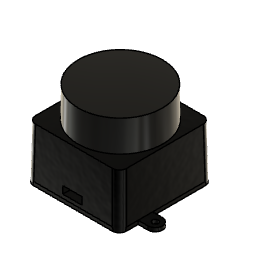
LD19激光雷达 v2 (Autodesk Fusion 360 design; units mm, degrees)
Autodesk Fusion 360 part; units mm, degrees
sketch "草图1" plane through (0, 0, 0) normal (0, 0, 1) x (1, 0, 0)
  line L0 (0, 0) -> (38.59, 0)
  line L1 (38.59, 0) -> (38.59, 38.59)
  line L2 (38.59, 38.59) -> (0, 38.59)
  line L3 (0, 38.59) -> (0, 0)
  line L4 (19.295, 40.7359) -> (19.295, -30)
  circle A0 centre (-4.105, 10.78) radius 1.25
  circle A1 centre (-4.105, 10.78) radius 3
  circle A2 centre (42.695, 10.78) radius 1.25
  circle A3 centre (42.695, 10.78) radius 3
  circle A4 centre (19.3, 42.7) radius 1.25
  circle A5 centre (19.3, 42.7) radius 3
  line L5 (16.3, 38.59) -> (22.3, 38.59)
  line L6 (22.3, 38.59) -> (22.3, 42.7)
  line L7 (16.3, 42.7) -> (16.3, 38.59)
  line L8 (38.59, 13.78) -> (42.695, 13.78)
  line L9 (42.695, 7.78) -> (38.59, 7.78)
  line L10 (38.59, 7.78) -> (38.59, 13.78)
  line L11 (0, 13.78) -> (-4.105, 13.78)
  line L12 (-4.105, 7.78) -> (0, 7.78)
  line L13 (0, 7.78) -> (0, 13.78)
  dimension "d1" = 38.59
  dimension "d2" = 38.59
  dimension "d3" = 2.5
  dimension "d4" = 6
  dimension "d5" = 46.8
  dimension "d6" = 27.81
  dimension "d7" = 2.5
  dimension "d8" = 6
  dimension "d9" = 19.29
  dimension "d10" = 31.92
  constraint horizontal L0
  constraint vertical L1
  constraint horizontal L2
  constraint vertical L3
  constraint coincident L0.start L3.end
  constraint perpendicular L2 L4
  constraint concentric A0 A1
  constraint symmetric L4 A0 A2
  constraint symmetric L4 A1 A3
  constraint concentric A4 A5
  constraint horizontal L5
  constraint vertical L6
  constraint vertical L7
  constraint coincident L2 L5.start
  constraint tangent A5 L7
  constraint tangent A5 L6
  constraint coincident A5 L6.end
  constraint coincident A5 L7.start
  constraint horizontal L8
  constraint horizontal L9
  constraint vertical L10
  constraint coincident L1 L8.start
  constraint tangent A3 L8
  constraint tangent A3 L9
  constraint coincident A3 L8.end
  constraint coincident A3 L9.start
  constraint horizontal L11
  constraint horizontal L12
  constraint vertical L13
  constraint coincident L3 L11.start
  constraint tangent A1 L11
  constraint tangent A1 L12
  constraint coincident A1 L11.end
  constraint coincident A1 L12.start
  measures "d1" distance of L1.end L2.end
  measures "d2" distance of L0.start L2.end
  measures "d3" diameter of A0
  measures "d4" diameter of A1
  measures "d5" distance of A0.centre A2.centre
  measures "d6" distance of L2 A2.centre
  measures "d7" diameter of A4
  measures "d8" diameter of A5
  measures "d9" distance of L1 A4.centre
  measures "d10" vertical distance of A2.centre A4.centre
extrude "拉伸1" add sketch "草图1" along normal blind 1.5 makes body 1
sketch "草图2" plane through (0, 0, 1.5) normal (0, 0, 1) x (-1, 0, 0)
  circle A0 centre (-42.695, -10.78) radius 1.25
  circle A1 centre (4.105, -10.78) radius 1.25
  circle A2 centre (-19.3, -42.7) radius 1.25
  line L0 (-38.59, -13.78) -> (-38.59, -38.59)
  line L1 (-38.59, -38.59) -> (-22.3, -38.59)
  line L2 (-22.3, -38.59) -> (-22.3, -42.7)
  arc A3 (-22.3, -42.7) -> (-16.3, -42.7) centre (-19.3, -42.7) ccw
  line L3 (-16.3, -42.7) -> (-16.3, -38.59)
  line L4 (-16.3, -38.59) -> (0, -38.59)
  line L5 (0, -38.59) -> (0, -13.78)
  line L6 (0, -13.78) -> (4.105, -13.78)
  arc A4 (4.105, -13.78) -> (4.105, -7.78) centre (4.105, -10.78) ccw
  line L7 (4.105, -7.78) -> (0, -7.78)
  line L8 (0, -7.78) -> (0, 0)
  line L9 (0, 0) -> (-38.59, 0)
  line L10 (-38.59, 0) -> (-38.59, -7.78)
  line L11 (-38.59, -7.78) -> (-42.695, -7.78)
  arc A5 (-42.695, -7.78) -> (-42.695, -13.78) centre (-42.695, -10.78) ccw
  line L12 (-42.695, -13.78) -> (-38.59, -13.78)
  line L13 (0, 0) -> (-38.59, 0)
  line L14 (-38.59, 0) -> (-38.59, -38.59)
  line L15 (-38.59, -38.59) -> (0, -38.59)
  line L16 (0, -38.59) -> (0, 0)
  constraint horizontal L13
  constraint vertical L14
  constraint horizontal L15
  constraint vertical L16
  constraint coincident L0.end L1.start
  constraint coincident L8.end L9.start
extrude "拉伸2" add sketch "草图2" along normal blind 20.7 draft -1 contours L0 L1 L4 L5 L8 L9 L10 L13 L14 L15 L16 bodies 1
fillet "圆角1" radius 3 1 edges at (0.1807, 0.1807, 11.85) on bodies 1
fillet "圆角2" radius 3 3 edges at (38.4093, 0.1807, 11.85) (38.4093, 38.4093, 11.85) (0.1807, 38.4093, 11.85) on bodies 1
sketch "草图3" plane through (0, 0, 22.2) normal (0, 0, 1) x (-1, 0, 0)
  ellipse E0 centre (-3.3618, -35.2282) end of major axis (-1.2398, -37.3502) minor radius 3 (-3.3609, -38.2287) -> (-0.3613, -35.2291) ccw
  line L0 (-0.3613, -35.2291) -> (-0.3613, -3.3609)
  ellipse E1 centre (-3.3618, -3.3618) end of major axis (-1.2398, -1.2398) minor radius 3 (-0.3613, -3.3609) -> (-3.3609, -0.3613) ccw
  line L1 (-3.3609, -0.3613) -> (-35.2291, -0.3613)
  ellipse E2 centre (-35.2282, -3.3618) end of major axis (-37.3502, -1.2398) minor radius 3 (-35.2291, -0.3613) -> (-38.2287, -3.3609) ccw
  line L2 (-38.2287, -3.3609) -> (-38.2287, -35.2291)
  ellipse E3 centre (-35.2282, -35.2282) end of major axis (-37.3502, -37.3502) minor radius 3 (-38.2287, -35.2291) -> (-35.2291, -38.2287) ccw
  line L3 (-35.2291, -38.2287) -> (-3.3609, -38.2287)
  circle A0 centre (-19.3478, -19.6362) radius 17.645
  dimension "d19" = 35.29
  measures "d19" diameter of A0
extrude "拉伸3" add sketch "草图3" along normal blind 12.8 draft -1 separate body contours A0 makes body 2
sketch "草图4" plane through (0, -0.0262, 0.0005) normal (0, -0.999848, 0.017452) x (1, 0, 0)
  line L0 (35.5905, 1.4998) -> (35.2291, 22.2029)
  line L1 (35.2291, 22.2029) -> (3.3609, 22.2029)
  line L2 (3.3609, 22.2029) -> (2.9995, 1.4998)
  line L3 (2.9995, 1.4998) -> (35.5905, 1.4998)
  line L4 (15, 6) -> (23, 6)
  line L5 (23, 6) -> (23, 3)
  line L6 (23, 3) -> (15, 3)
  line L7 (15, 3) -> (15, 6)
  constraint horizontal L4
  constraint vertical L5
  constraint horizontal L6
  constraint vertical L7
extrude "拉伸4" cut sketch "草图4" against normal blind 4 contours L4 L5 L6 L7 bodies 1
copy_body "实体->零部件1" bodies 1 removing the originals makes body 3 in component "Component'"
copy_body "实体->零部件2" bodies 2 removing the originals makes body 4 in component "Component''"
component "Component'" placed x (1, 0, 0) y (0, 1, 0) z (0, 0, 1) at (0, 0, 0)
component "Component''" placed x (1, 0, 0) y (0, 1, 0) z (0, 0, 1) at (0, 0, 0)
